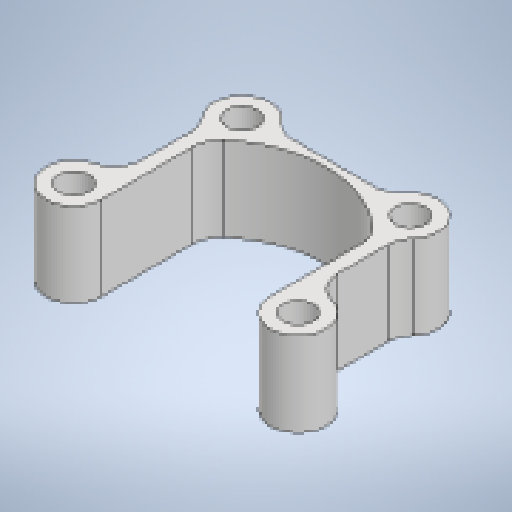
# Autodesk Inventor part: Chassis
Saved by Autodesk Inventor 2023.1 (Build 271208000, 208)
## iProperties
Created: 2022-08-25
Part Number: Chassis
Material: Generic
Document SubType Name: Modeling
Designer: Nathan Cai
Density: 1 g/cm^3
Appearance: Default
Author: Nathan Cai
Autodesk Inventor part; units mm, degrees
ref_plane "YZ Plane" through (0, 0, 0) normal (1, 0, 0) x (0, 1, 0)
ref_plane "XZ Plane" through (0, 0, 0) normal (0, 1, 0) x (-1, 0, 0)
ref_plane "XY Plane" through (0, 0, 0) normal (0, 0, 1) x (1, 0, 0)
sketch "Sketch1" plane through (0, 0, 0) normal (0, 1, 0) x (-1, 0, 0)
  circle A0 centre (26.9875, 31.75) radius 3.429
  line L0 (0, 0) -> (0, -38.1) construction
  circle A1 centre (26.9875, 31.75) radius 6.35
  line L1 (0, 0) -> (20.6375, 0) construction
  line L2 (20.6375, 31.75) -> (0, 31.75) construction
  line L3 (0, 31.75) -> (0, 0) construction
  circle A2 centre (20.6375, 0) radius 3.429
  circle A3 centre (20.6375, 0) radius 6.35
  line L4 (20.6375, 6.35) -> (20.6375, 31.75)
  line L5 (23.8125, 26.2507) -> (23.8125, 5.4993)
  arc A4 (0, 0) -> (20.6375, 8.0926) centre (0, 30.3609) ccw
  line L6 (0, 0) -> (20.6375, 0)
  line L7 (0, -1.5875) -> (14.4891, -1.5875)
  circle A5 centre (-26.9875, 31.75) radius 3.429
  circle A6 centre (-26.9875, 31.75) radius 6.35
  line L8 (0, 0) -> (-20.6375, 0) construction
  line L9 (-20.6375, 31.75) -> (0, 31.75) construction
  circle A7 centre (-20.6375, 0) radius 3.429
  circle A8 centre (-20.6375, 0) radius 6.35
  line L10 (-20.6375, 6.35) -> (-20.6375, 31.75)
  line L11 (-23.8125, 26.2507) -> (-23.8125, 5.4993)
  arc A9 (-20.6375, 8.0926) -> (0, 0) centre (0, 30.3609) ccw
  line L12 (0, 0) -> (-20.6375, 0)
  line L13 (0, -1.5875) -> (-14.4891, -1.5875)
  dimension "d0" = 6.858
  dimension "d1" = 38.1
  dimension "d2" = 26.9875
  dimension "d3" = 12.7
  dimension "d5" = 31.75
  dimension "d9" = 6.858
  dimension "d10" = 12.7
  dimension "d11" = 3.175
  dimension "d13" = 1.5875
  constraints: 28 end point, 14 point on circle, 11 symmetric about line, 10 centre point, 6 coincident, 4 parallel, 4 point on line, 3 tangent, 1 collinear, 1 horizontal, 1 perpendicular, 1 vertical, 5 other
  measures "d0" diameter of A0
  measures "d1" distance of L0.start L0.end
  measures "d2" distance from line of A0.centre L0
  measures "d3" diameter of A1
  measures "d5" distance between parallel lines of L1 L2
  measures "d9" diameter of A2
  measures "d10" diameter of A3
  measures "d11" distance between parallel lines of L4 L5
  measures "d13" distance between parallel lines of L1 L7
extrude "Extrusion1" add sketch "Sketch1" along normal blind 19.05
fillet "Fillet1" radius 6.35 8 edges at (-20.6375, 9.525, 8.0926) (20.6375, 9.525, 8.0926) (-14.4891, 9.525, -1.5875) (14.4891, 9.525, -1.5875) (23.8125, 9.525, 5.4993) (23.8125, 9.525, 26.2507) (-23.8125, 9.525, 5.4993) (-23.8125, 9.525, 26.2507)
body "Solid1"
